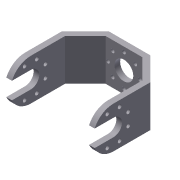
# Autodesk Inventor part: Waistline
Saved by Autodesk Inventor 2011 (Build 150239000, 239)
## iProperties
Created: 2010-11-22
Part Number: Waistline
Document SubType Name: Modeling
Designer: Milton
Density: 2.71 g/cm^3
Mass: 16.2054 g
Surface Area: 53.6309 cm^2
Volume: 5.97984 cm^3
Material: Aluminum-6061
Author: Milton
Autodesk Inventor part; units mm, degrees
ref_plane "YZ Plane" through (0, 0, 0) normal (1, 0, 0) x (0, 1, 0)
ref_plane "XZ Plane" through (0, 0, 0) normal (0, 1, 0) x (-1, 0, 0)
ref_plane "XY Plane" through (0, 0, 0) normal (0, 0, 1) x (1, 0, 0)
sketch "Sketch1" plane through (0, 0, 0) normal (0, 0, 1) x (1, 0, 0)
  line L0 (-20.5, -40) -> (-20.5, -10.7426)
  line L1 (-9.7574, 0) -> (9.7574, 0)
  line L2 (20.5, -10.7426) -> (20.5, -40)
  line L3 (20.5, -40) -> (23.5, -40)
  line L4 (23.5, -40) -> (23.5, -9.5)
  line L5 (-20.5, -40) -> (-23.5, -40)
  line L6 (-23.5, -40) -> (-23.5, -9.5)
  line L7 (-11, 3) -> (11, 3)
  line L8 (-11, 3) -> (-23.5, -9.5)
  line L9 (-9.7574, 0) -> (-20.5, -10.7426)
  line L10 (11, 3) -> (23.5, -9.5)
  line L11 (9.7574, 0) -> (20.5, -10.7426)
  point P0 (0, 0)
  constraints: 24 end point
extrude "Extrusion1" add sketch "Sketch1" along normal blind 22
sketch "Sketch2" plane through (23.5, -40, 0) normal (1, 0, 0) x (0, 0, -1)
  line L0 (-22, 30.5) -> (-22, 0) projected
  line L1 (0, 0) -> (-22, 0) projected
  line L2 (0, 0) -> (0, 30.5) projected
  line L3 (0, 30.5) -> (-22, 30.5) projected
  arc A0 (-22, 11) -> (0, 11) centre (-11, 11) ccw
  line L4 (-22, 29.2574) -> (-22, 0) projected
  line L5 (-22, 11) -> (-22, -1)
  line L6 (-22, -1) -> (0, -1)
  line L7 (0, -1) -> (0, 11)
  line L8 (0, 0) -> (0, 29.2574) projected
  circle A1 centre (-11, 11) radius 4.5
  line L9 (-15.5, 11) -> (-15.5, -1)
  line L10 (-6.5, 11) -> (-6.5, -1)
  point P0 (0, 40)
  dimension "d2" = 22
  dimension "d3" = 11
  dimension "d4" = 9
  constraints: 10 end point, 4 point on circle, 4 point on line, 3 perpendicular, 3 tangent, 2 centre point, 1 coincident, 1 collinear
  measures "d2" diameter of A0
  measures "d3" distance from line of L1 A0.centre
  measures "d4" diameter of A1
extrude "Extrusion2" cut sketch "Sketch2" against normal through all contours A0 L9 L1 L0 | L1 L9 L6 L5 | L9 A1 L10 A0 | A0 L1 L9 | L2 L1 L10 A0 | L1 L10 L6 L9 | A0 L10 L1 | A1 | L7 L6 L10 L1
sketch "Sketch3" plane through (-9.7574, 0, 0) normal (0, -1, 0) x (1, 0, 0)
  circle A0 centre (9.7574, 11) radius 5
  point P0 (9.7574, 0)
  dimension "d7" = 10
  constraints: 1 centre point
  measures "d7" diameter of A0
extrude "Extrusion3" cut sketch "Sketch3" against normal through all
sketch "Sketch4" plane through (23.5, -9.5, 22) normal (1, 0, 0) x (0, 0, -1)
  arc A0 (15.5, -29.5374) -> (22, -19.5) centre (11, -19.5) ccw projected
  line L0 (11, -19.5) -> (18.853, -16.2472)
  line L1 (11, -19.5) -> (19.5, -19.5) construction
  circle A1 centre (18.853, -16.2472) radius 1
  point P0 (22, 9.5)
  dimension "d10" = 8.5
  dimension "d11" = 22.5
  dimension "d12" = 2
  constraints: 4 end point, 1 centre point, 1 coincident, 1 equal length, 1 horizontal
  measures "d10" distance of L0.start L0.end
  measures "d11" angle of L1 L0
  measures "d12" diameter of A1
extrude "Extrusion4" cut sketch "Sketch4" against normal through all
pattern_circular "Circular Pattern1" count 8 over 360 about axis through (23.5, -29, 11) along (-1, 0, 0) of "Extrusion4"
sketch "Sketch5" plane through (-9.7574, 0, 0) normal (0, -1, 0) x (1, 0, 0)
  circle A0 centre (9.7574, 11) radius 5 projected
  circle A1 centre (9.7574, 19.5) radius 1
  point P0 (9.7574, 0)
  dimension "d18" = 2
  dimension "d19" = 8.5
  constraints: 1 centre point
  measures "d18" diameter of A1
  measures "d19" distance of A0.centre A1.centre
extrude "Extrusion5" cut sketch "Sketch5" against normal through all contours A1
pattern_circular "Circular Pattern2" count 8 over 360 about axis through (0, 0, 11) along (0, 1, 0) of "Extrusion5"
body "Solid1"
